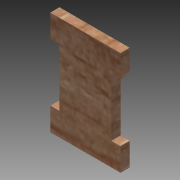
# Autodesk Inventor part: tussenplaatje
Saved by Autodesk Inventor 2015 (Build 190159000, 159)
## iProperties
Created: 2016-01-23
Part Number: tussenplaatje
Material: Generic
Document SubType Name: Modeling
Designer: david
Density: 1 g/cm^3
Appearance: Birch - Natural Polished
Author: david
Autodesk Inventor part; units mm, degrees
ref_plane "YZ Plane" through (0, 0, 0) normal (1, 0, 0) x (0, 1, 0)
ref_plane "XZ Plane" through (0, 0, 0) normal (0, 1, 0) x (-1, 0, 0)
ref_plane "XY Plane" through (0, 0, 0) normal (0, 0, 1) x (1, 0, 0)
sketch "Sketch1" plane through (0, 0, 0) normal (0, 1, 0) x (-1, 0, 0)
  line L0 (-7.25, 20) -> (7.25, 20)
  line L1 (7.25, 20) -> (7.25, -20)
  line L2 (7.25, -20) -> (-7.25, -20)
  line L3 (-7.25, -20) -> (-7.25, 20)
  line L4 (-7.25, 20) -> (7.25, -20) construction
  line L5 (7.25, 20) -> (-7.25, -20) construction
  point P0 (0, 0)
  dimension "d0" = 14.5
  dimension "d1" = 40
  constraints: 12 end point, 2 midpoint, 2 parallel, 1 horizontal, 1 perpendicular
  measures "d0" distance of L1.end L2.end
  measures "d1" distance of L0.end L1.end
extrude "Extrusion1" add sketch "Sketch1" along normal blind 4
sketch "Sketch2" plane through (0, 4, 0) normal (0, 1, 0) x (1, 0, 0)
  line L0 (7.25, -20) -> (11.25, -20)
  line L1 (11.25, -20) -> (11.25, -10)
  line L2 (11.25, -10) -> (7.25, -10)
  line L3 (7.25, -10) -> (7.25, -20)
  line L4 (7.25, 20) -> (11.25, 20)
  line L5 (11.25, 20) -> (11.25, 10)
  line L6 (11.25, 10) -> (7.25, 10)
  line L7 (7.25, 10) -> (7.25, 20)
  line L8 (0, -21.4425) -> (0, 24.9563)
  line L9 (-7.25, -20) -> (-11.25, -20)
  line L10 (-11.25, -20) -> (-11.25, -10)
  line L11 (-11.25, -10) -> (-7.25, -10)
  line L12 (-7.25, -10) -> (-7.25, -20)
  line L13 (-7.25, 20) -> (-11.25, 20)
  line L14 (-11.25, 20) -> (-11.25, 10)
  line L15 (-11.25, 10) -> (-7.25, 10)
  line L16 (-7.25, 10) -> (-7.25, 20)
  point P0 (0, 0)
  point P1 (-11.25, -20)
  point P2 (-11.25, 20)
  dimension "d4" = 4
  dimension "d5" = 10
  dimension "d6" = 4
  dimension "d7" = 10
  constraints: 34 end point, 8 symmetric about line, 4 parallel, 2 horizontal, 2 perpendicular, 1 vertical
  measures "d4" distance of L2.end L1.end
  measures "d5" distance of L1.end L0.end
  measures "d6" distance of L5.end L6.end
  measures "d7" distance of L4.end L5.end
extrude "Extrusion2" add sketch "Sketch2" against normal blind 4
body "Solid1"
